Autodesk Inventor part; units mm, degrees
(part 2 of 2)
sketch "Sketch5" plane through (-17.4625, 17.4625, -76.2) normal (0, 0, -1) x (-1, 0, 0)
  line L0 (0, 66.675) -> (0, 0)
  line L1 (0, 33.3375) -> (41.275, 33.3375)
  line L2 (41.275, 0) -> (41.275, 66.675)
  line L3 (2.8791, 33.3375) -> (-5.5086, 33.3375)
  line L4 (-5.5086, 33.3375) -> (-5.5086, 35.5502)
  line L5 (-5.5086, 35.5502) -> (-2.8328, 35.5502)
  line L6 (-2.8328, 35.5502) -> (-2.8328, 42.2707)
  line L7 (-2.8328, 42.2707) -> (-5.5086, 42.2707)
  line L8 (-5.5086, 42.2707) -> (-5.5086, 44.3394)
  spline S0 degree 2 poles (-5.5086, 44.3394) (-4.922, 44.3394) (-3.7591, 44.4937) (-3.4091, 44.6584) knots 0 0 0 1 2 2 2
  spline S1 degree 2 poles (-3.4091, 44.6584) (-3.0078, 44.8642) (-2.5549, 45.5538) (-2.5138, 46.0684) knots 0 0 0 1 2 2 2
  line L9 (-2.5138, 46.0684) -> (0.265, 46.0684)
  line L10 (0.265, 46.0684) -> (0.265, 35.5502)
  line L11 (0.265, 35.5502) -> (2.8791, 35.5502)
  line L12 (2.8791, 35.5502) -> (2.8791, 33.3375)
  spline S2 degree 2 poles (14.2515, 37.1866) (14.2515, 36.2501) (13.5619, 34.7166) (12.893, 34.1814) knots 0 0 0 1 2 2 2
  spline S3 degree 2 poles (12.893, 34.1814) (12.224, 33.6463) (10.4024, 33.0699) (9.0953, 33.0699) knots 0 0 0 1 2 2 2
  spline S4 degree 2 poles (9.0953, 33.0699) (7.6133, 33.0699) (5.4932, 33.5639) (4.8243, 33.8727) knots 0 0 0 1 2 2 2
  line L13 (4.8243, 33.8727) -> (4.8243, 36.6309)
  line L14 (4.8243, 36.6309) -> (5.133, 36.6309)
  spline S5 degree 2 poles (5.133, 36.6309) (5.8328, 36.1883) (7.7162, 35.5296) (8.4984, 35.5296) knots 0 0 0 1 2 2 2
  spline S6 degree 2 poles (8.4984, 35.5296) (8.9615, 35.5296) (10.0422, 35.6943) (10.4127, 35.9619) knots 0 0 0 1 2 2 2
  spline S7 degree 2 poles (10.4127, 35.9619) (10.7008, 36.178) (11.0508, 36.8058) (11.0508, 37.3719) knots 0 0 0 1 2 2 2
  spline S8 degree 2 poles (11.0508, 37.3719) (11.0508, 37.9379) (10.5567, 38.5451) (10.1451, 38.6892) knots 0 0 0 1 2 2 2
  spline S9 degree 2 poles (10.1451, 38.6892) (9.7334, 38.8333) (8.591, 38.8642) (8.1485, 38.8642) knots 0 0 0 1 2 2 2
  line L15 (8.1485, 38.8642) -> (7.603, 38.8642)
  line L16 (7.603, 38.8642) -> (7.603, 41.0975)
  line L17 (7.603, 41.0975) -> (8.1073, 41.0975)
  spline S10 degree 2 poles (8.1073, 41.0975) (8.6837, 41.0975) (9.6614, 41.2004) (10.001, 41.3548) knots 0 0 0 1 2 2 2
  spline S11 degree 2 poles (10.001, 41.3548) (10.3406, 41.5194) (10.7214, 42.0958) (10.7214, 42.5898) knots 0 0 0 1 2 2 2
  spline S12 degree 2 poles (10.7214, 42.5898) (10.7214, 42.9809) (10.3612, 43.4646) (10.1039, 43.5984) knots 0 0 0 1 2 2 2
  spline S13 degree 2 poles (10.1039, 43.5984) (9.7952, 43.7527) (8.9718, 43.8557) (8.6837, 43.8557) knots 0 0 0 1 2 2 2
  spline S14 degree 2 poles (8.6837, 43.8557) (8.2205, 43.8557) (7.2428, 43.6395) (6.79, 43.4646) knots 0 0 0 1 2 2 2
  spline S15 degree 2 poles (6.79, 43.4646) (6.4298, 43.3308) (5.6476, 42.8985) (5.4623, 42.7853) knots 0 0 0 1 2 2 2
  line L18 (5.4623, 42.7853) -> (5.1948, 42.7853)
  line L19 (5.1948, 42.7853) -> (5.1948, 45.5023)
  spline S16 degree 2 poles (5.1948, 45.5023) (5.8534, 45.7802) (8.0764, 46.3051) (9.2394, 46.3051) knots 0 0 0 1 2 2 2
  spline S17 degree 2 poles (9.2394, 46.3051) (10.3715, 46.3051) (12.0388, 45.914) (12.6254, 45.5332) knots 0 0 0 1 2 2 2
  spline S18 degree 2 poles (12.6254, 45.5332) (13.2738, 45.1318) (13.9221, 43.8968) (13.9221, 43.1249) knots 0 0 0 1 2 2 2
  spline S19 degree 2 poles (13.9221, 43.1249) (13.9221, 42.034) (12.6666, 40.4079) (11.6374, 40.1712) knots 0 0 0 1 2 2 2
  line L20 (11.6374, 40.1712) -> (11.6374, 40.0477)
  spline S20 degree 2 poles (11.6374, 40.0477) (12.0902, 39.986) (12.9547, 39.6566) (13.3664, 39.2861) knots 0 0 0 1 2 2 2
  spline S21 degree 2 poles (13.3664, 39.2861) (13.7472, 38.9568) (14.2515, 37.907) (14.2515, 37.1866) knots 0 0 0 1 2 2 2
  spline S22 degree 2 poles (25.665, 36.8676) (25.665, 36.0545) (24.9858, 34.6446) (24.3374, 34.13) knots 0 0 0 1 2 2 2
  spline S23 degree 2 poles (24.3374, 34.13) (23.689, 33.6154) (21.8262, 33.039) (20.6221, 33.039) knots 0 0 0 1 2 2 2
  spline S24 degree 2 poles (20.6221, 33.039) (19.3356, 33.039) (17.411, 33.6257) (16.7935, 34.13) knots 0 0 0 1 2 2 2
  spline S25 degree 2 poles (16.7935, 34.13) (16.1863, 34.6343) (15.61, 36.0031) (15.61, 36.7646) knots 0 0 0 1 2 2 2
  spline S26 degree 2 poles (15.61, 36.7646) (15.61, 37.8556) (16.8141, 39.3067) (17.9565, 39.7904) knots 0 0 0 1 2 2 2
  line L21 (17.9565, 39.7904) -> (17.9565, 39.8419)
  spline S27 degree 2 poles (17.9565, 39.8419) (16.8347, 40.3873) (15.9496, 41.9414) (15.9496, 42.8985) knots 0 0 0 1 2 2 2
  spline S28 degree 2 poles (15.9496, 42.8985) (15.9496, 43.5984) (16.5671, 44.8231) (17.1743, 45.3068) knots 0 0 0 1 2 2 2
  spline S29 degree 2 poles (17.1743, 45.3068) (17.761, 45.7699) (19.5414, 46.3257) (20.6529, 46.3257) knots 0 0 0 1 2 2 2
  spline S30 degree 2 poles (20.6529, 46.3257) (21.8262, 46.3257) (23.5758, 45.8214) (24.1418, 45.4097) knots 0 0 0 1 2 2 2
  spline S31 degree 2 poles (24.1418, 45.4097) (24.7182, 44.998) (25.3357, 43.8042) (25.3357, 43.1146) knots 0 0 0 1 2 2 2
  spline S32 degree 2 poles (25.3357, 43.1146) (25.3357, 42.209) (24.2859, 40.7578) (23.2053, 40.2535) knots 0 0 0 1 2 2 2
  line L22 (23.2053, 40.2535) -> (23.2053, 40.2124)
  spline S33 degree 2 poles (23.2053, 40.2124) (24.4712, 39.6978) (25.665, 38.0305) (25.665, 36.8676) knots 0 0 0 1 2 2 2
  spline S34 degree 2 poles (22.5157, 36.7338) (22.5157, 37.3616) (21.9806, 38.0202) (21.1161, 38.4422) knots 0 0 0 1 2 2 2
  spline S35 degree 2 poles (21.1161, 38.4422) (20.8691, 38.5554) (19.9325, 38.9156) (19.5723, 39.07) knots 0 0 0 1 2 2 2
  spline S36 degree 2 poles (19.5723, 39.07) (19.243, 38.7407) (18.7181, 37.7527) (18.7181, 37.166) knots 0 0 0 1 2 2 2
  spline S37 degree 2 poles (18.7181, 37.166) (18.7181, 36.2809) (19.8502, 35.2209) (20.7661, 35.2209) knots 0 0 0 1 2 2 2
  spline S38 degree 2 poles (20.7661, 35.2209) (21.0234, 35.2209) (21.6615, 35.3856) (21.9085, 35.5502) knots 0 0 0 1 2 2 2
  spline S39 degree 2 poles (21.9085, 35.5502) (22.1864, 35.7458) (22.5157, 36.2809) (22.5157, 36.7338) knots 0 0 0 1 2 2 2
  spline S40 degree 2 poles (22.2379, 42.7441) (22.2379, 43.3925) (21.3837, 44.1644) (20.6529, 44.1644) knots 0 0 0 1 2 2 2
  spline S41 degree 2 poles (20.6529, 44.1644) (19.9531, 44.1644) (19.0989, 43.4646) (19.0989, 42.95) knots 0 0 0 1 2 2 2
  spline S42 degree 2 poles (19.0989, 42.95) (19.0989, 42.4457) (19.6135, 41.8179) (20.1589, 41.5606) knots 0 0 0 1 2 2 2
  spline S43 degree 2 poles (20.1589, 41.5606) (20.3956, 41.4371) (21.0543, 41.1798) (21.5998, 40.974) knots 0 0 0 1 2 2 2
  spline S44 degree 2 poles (21.5998, 40.974) (21.9291, 41.4062) (22.2379, 42.2193) (22.2379, 42.7441) knots 0 0 0 1 2 2 2
  line L23 (36.8213, 33.3375) -> (27.4866, 33.3375)
  line L24 (27.4866, 33.3375) -> (27.4866, 35.4061)
  spline S45 degree 2 poles (27.4866, 35.4061) (28.6702, 36.353) (30.5639, 38.0202) (31.274, 38.7715) knots 0 0 0 1 2 2 2
  spline S46 degree 2 poles (31.274, 38.7715) (32.2106, 39.7493) (33.0442, 41.2416) (33.0442, 42.0237) knots 0 0 0 1 2 2 2
  spline S47 degree 2 poles (33.0442, 42.0237) (33.0442, 42.9088) (31.9841, 43.8557) (31.0373, 43.8557) knots 0 0 0 1 2 2 2
  spline S48 degree 2 poles (31.0373, 43.8557) (30.5536, 43.8557) (29.6891, 43.6189) (29.2465, 43.4337) knots 0 0 0 1 2 2 2
  spline S49 degree 2 poles (29.2465, 43.4337) (28.8143, 43.2381) (28.1968, 42.8265) (28.0424, 42.7236) knots 0 0 0 1 2 2 2
  line L25 (28.0424, 42.7236) -> (27.7954, 42.7236)
  line L26 (27.7954, 42.7236) -> (27.7954, 45.492)
  spline S50 degree 2 poles (27.7954, 45.492) (28.3306, 45.7493) (30.6153, 46.2845) (31.6754, 46.2845) knots 0 0 0 1 2 2 2
  spline S51 degree 2 poles (31.6754, 46.2845) (33.9396, 46.2845) (36.2655, 44.2673) (36.2655, 42.4457) knots 0 0 0 1 2 2 2
  spline S52 degree 2 poles (36.2655, 42.4457) (36.2655, 41.3239) (35.2054, 39.1626) (33.9807, 37.9276) knots 0 0 0 1 2 2 2
  spline S53 degree 2 poles (33.9807, 37.9276) (33.2089, 37.166) (31.7577, 35.9825) (31.4387, 35.7355) knots 0 0 0 1 2 2 2
  line L27 (31.4387, 35.7355) -> (36.8213, 35.7355)
  line L28 (36.8213, 35.7355) -> (36.8213, 33.3375)
  line L29 (47.9466, 33.3375) -> (38.612, 33.3375)
  line L30 (38.612, 33.3375) -> (38.612, 35.4061)
  spline S54 degree 2 poles (38.612, 35.4061) (39.7956, 36.353) (41.6892, 38.0202) (42.3994, 38.7715) knots 0 0 0 1 2 2 2
  spline S55 degree 2 poles (42.3994, 38.7715) (43.3359, 39.7493) (44.1695, 41.2416) (44.1695, 42.0237) knots 0 0 0 1 2 2 2
  spline S56 degree 2 poles (44.1695, 42.0237) (44.1695, 42.9088) (43.1095, 43.8557) (42.1627, 43.8557) knots 0 0 0 1 2 2 2
  spline S57 degree 2 poles (42.1627, 43.8557) (41.6789, 43.8557) (40.8144, 43.6189) (40.3719, 43.4337) knots 0 0 0 1 2 2 2
  spline S58 degree 2 poles (40.3719, 43.4337) (39.9396, 43.2381) (39.3221, 42.8265) (39.1678, 42.7236) knots 0 0 0 1 2 2 2
  line L31 (39.1678, 42.7236) -> (38.9208, 42.7236)
  line L32 (38.9208, 42.7236) -> (38.9208, 45.492)
  spline S59 degree 2 poles (38.9208, 45.492) (39.4559, 45.7493) (41.7407, 46.2845) (42.8007, 46.2845) knots 0 0 0 1 2 2 2
  spline S60 degree 2 poles (42.8007, 46.2845) (45.0649, 46.2845) (47.3909, 44.2673) (47.3909, 42.4457) knots 0 0 0 1 2 2 2
  spline S61 degree 2 poles (47.3909, 42.4457) (47.3909, 41.3239) (46.3308, 39.1626) (45.1061, 37.9276) knots 0 0 0 1 2 2 2
  spline S62 degree 2 poles (45.1061, 37.9276) (44.3342, 37.166) (42.8831, 35.9825) (42.564, 35.7355) knots 0 0 0 1 2 2 2
  line L33 (42.564, 35.7355) -> (47.9466, 35.7355)
  line L34 (47.9466, 35.7355) -> (47.9466, 33.3375)
  point P0 (58.7375, -17.4625)
  point P1 (58.7375, -17.4625)
  constraints: 6 end point, 2 midpoint, 1 horizontal
extrude "Extrusion4" cut sketch "Sketch4" against normal blind 5.08 contours S10 S7 L3 L0 S17 S18 S11 S12 | L0 S12 S13 S14 S15 S16 S17 S7 S8 S9 S10 | S7 L0 L3 | S52 S53 L1 | L1 S53 S54 S55 L67 L68 L69 S44 S45 S46 L64 L65 S47 S48 S49 S50 L66 S51 S52 | L17 L18 L19 S21 S22 S19 L3 S20 L15 | L3 S19 S20 | L23 L24 L25 L26 L27 L21 L3 | L29 L30 L31 L3 | L41 L42 L43 L44 L45 L46 L47 L3 L37 L38 L39 | L49 L50 L51 L3 | L60 L61 L62 S42 S43 L63 L3 L57 S39 S40 S41 L58 | S28 S29 S30 S27 L3 | L3 S27 S28 | L4 L5 L6 L7 L8 L9 L10 S0 S1 S2 L11 | L32 L33 L34 L35 | L52 L53 L54 L55 | S61 L71 L72 S62 S63 S64 S65 S66 S67 S68 S69 S70 L73 L74 S71 S72 S73 S74 S75 S76 S77 S78
extrude "Extrusion5" cut sketch "Sketch5" against normal blind 5.08 contours L9 L10 L11 L12 L1 L0 | L0 L3 L4 L5 L6 L7 L8 S0 S1 L9 | L24 S45 S46 S47 S48 S49 L25 L26 S50 S51 S52 S53 L27 L28 L1 | L30 S54 L2 L1 | L2 S54 S55 S56 S57 S59 S60 S61 S62 L33 L34 L29 | S57 S58 L31 L32 S59 L2 | S4 L13 L14 S5 S6 S7 S8 S9 L15 L16 L17 S10 S11 S12 S13 S14 S15 L18 L19 S16 S17 S18 S19 L20 S20 S21 S2 S3 L1 | L1 S3 S4 | S24 S25 S26 L21 S27 S28 S29 S30 S31 S32 L22 S33 S22 S23 L1 | L1 S23 S24
body "Solid1"
